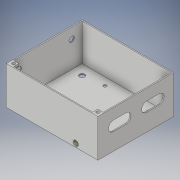
# Autodesk Inventor part: Caixa de Segurança_Sem fixação
Saved by Autodesk Inventor 2019 (Build 230136000, 136)
## iProperties
Created: 2020-05-23
Part Number: Caixa de Segurança_Sem fixação
Material: Genérico
Document SubType Name: Modeling
Designer: lukas
Density: 1 g/cm^3
Appearance: Padrão
Categories: <MemberInstance><Categories><Category DisplayName="" Mnemonic="CABLEANDHARNESS" InternalName="e4a7e005-5e42-4d16-b293-125e7f0d0512"><Category DisplayName="" Mnemonic="CONNECTORS" InternalName="6f634eba-a678-4820-a31d-2c2d5ee6728e"><CategoryParameter DisplayName="" Mnemonic="REFDES" InternalName="c3740e8c-60ab-4d5d-8584-52b73222f2f0"/><Category DisplayName="" Mnemonic="DISCRETEWIRE" InternalName="9a3407de-09b2-4cdb-8c40-9708d5144a28"/></Category></Category></Categories><FamilyTemplate><FamilyTemplateParameters></FamilyTemplateParameters></FamilyTemplate><CategoryParameterMap><ParamToTemplateMap><ParamToTemplate CategoryParameter="//CategoryParameter[@InternalName='c3740e8c-60ab-4d5d-8584-52b73222f2f0']" ConstantValue=""/></ParamToTemplateMap></CategoryParameterMap></MemberInstance>
Author: lukas
Autodesk Inventor part; units mm, degrees
ref_plane "YZ Plane" through (0, 0, 0) normal (1, 0, 0) x (0, 1, 0)
ref_plane "XZ Plane" through (0, 0, 0) normal (0, 1, 0) x (-1, 0, 0)
ref_plane "XY Plane" through (0, 0, 0) normal (0, 0, 1) x (1, 0, 0)
sketch "Esboço1" plane through (0, 0, 0) normal (0, 1, 0) x (-1, 0, 0)
  line L0 (-23.75, -30.48) -> (23.75, -30.48)
  line L1 (23.75, -30.48) -> (23.75, 30.48)
  line L2 (23.75, 30.48) -> (-23.75, 30.48)
  line L3 (-23.75, 30.48) -> (-23.75, -30.48)
  line L4 (-23.75, -30.48) -> (23.75, 30.48) construction
  line L5 (23.75, -30.48) -> (-23.75, 30.48) construction
  line L6 (-35, -35) -> (35, -35)
  line L7 (35, 35) -> (-35, 35)
  line L8 (-35, 35) -> (-35, -35)
  line L9 (-35, -35) -> (35, 35) construction
  line L10 (35, -35) -> (-35, 35) construction
  line L11 (23.75, 30.48) -> (20.75, 30.48)
  line L12 (23.75, 27.48) -> (23.75, 30.48)
  line L13 (-23.75, 30.48) -> (-20.75, 30.48)
  line L14 (-23.75, 27.48) -> (-23.75, 30.48)
  line L15 (-23.75, -30.48) -> (-20.75, -30.48)
  line L16 (-23.75, -27.48) -> (-23.75, -30.48)
  line L17 (23.75, -30.48) -> (20.75, -30.48)
  line L18 (23.75, -27.48) -> (23.75, -30.48)
  circle A0 centre (20.75, 27.48) radius 1.5
  circle A1 centre (-20.75, 27.48) radius 1.5
  circle A2 centre (-20.75, -27.48) radius 1.5
  circle A3 centre (20.75, -27.48) radius 1.5
  line L19 (35, -35) -> (50, -35)
  line L20 (50, -35) -> (50, 35)
  line L21 (50, 35) -> (35, 35)
  line L22 (50, -35) -> (40, -35)
  line L23 (40, -25) -> (40, 25)
  circle A4 centre (40, -25) radius 2.5
  circle A5 centre (40, 25) radius 2.5
  point P0 (0, 0)
  dimension "d0" = 47.5
  dimension "d1" = 60.96
  dimension "d12" = 3
  dimension "d13" = 3
  dimension "d33" = 15
  dimension "d34" = 70
  dimension "d35" = 10
  dimension "d36" = 10
  dimension "d37" = 50
  dimension "d38" = 5
  dimension "d39" = 5
  constraints: 48 end point, 6 centre point, 6 horizontal, 4 midpoint, 3 parallel, 3 perpendicular, 2 coincident, 2 point on line
  measures "d0" distance of L2.end L1.end
  measures "d1" distance of L1.end L0.end
  measures "d12" diameter of A1
  measures "d13" diameter of A2
  measures "d33" distance of L6.end L19.end
  measures "d34" distance of L19.end L20.end
  measures "d35" distance of L19.end L22.end
  measures "d36" distance of L22.end L23.start
  measures "d37" distance of L23.start L23.end
  measures "d38" diameter of A4
  measures "d39" diameter of A5
extrude "Extrusão1" add sketch "Esboço1" along normal blind 35 contours L3 L2 L1 L0 | L8 L7 L21 L20 L19 L6 | A4 | A5
shell "Casca1" thickness 1 outward yes removed faces 5 at (6.6326, 35, -8.7485) at (19.2549, 23.3333, 27.3593) at (-22.2451, 23.3333, -27.6007) at (-22.2451, 23.3333, 27.3593) at (19.2549, 23.3333, -27.6007)
sketch "Esboço3" plane through (-50, 0, -35) normal (0, 1, 0) x (1, 0, 0)
  line L0 (0, 0) -> (85, 0) projected
  line L1 (0, 0) -> (10, 0)
  line L2 (10, 0) -> (10, -10)
  line L3 (10, -10) -> (10, -60)
  circle A0 centre (10, -10) radius 2.5
  circle A1 centre (10, -60) radius 2.5
  point P0 (50, -35)
  dimension "d40" = 10
  dimension "d41" = 10
  dimension "d42" = 50
  dimension "d43" = 5
  dimension "d44" = 5
  constraints: 6 end point, 2 centre point, 2 coincident, 2 point on line, 1 vertical
  measures "d40" distance of L0.start L1.end
  measures "d41" distance of L1.end L2.end
  measures "d42" distance of L2.end L3.end
  measures "d43" diameter of A0
  measures "d44" diameter of A1
extrude "Extrusão3" cut sketch "Esboço3" against normal blind 1
sketch "Esboço4" plane through (-50, 0, -35) normal (1, 0, 0) x (0, 0, -1)
  line L0 (-70, 0) -> (-70, 35) projected
  line L1 (-70, 35) -> (-60, 35)
  line L2 (-70, 35) -> (0, 35) projected
  line L3 (-60, 35) -> (-60, 25)
  line L4 (0, 0) -> (0, 35) projected
  line L5 (0, 35) -> (-10, 35)
  line L6 (-10, 35) -> (-10, 25)
  circle A0 centre (-60, 25) radius 2.5
  circle A1 centre (-10, 25) radius 2.5
  point P0 (-35, 0)
  dimension "d47" = 10
  dimension "d48" = 10
  dimension "d49" = 10
  dimension "d50" = 10
  dimension "d51" = 5
  dimension "d52" = 5
  constraints: 8 end point, 2 centre point, 2 coincident, 2 perpendicular, 2 point on line
  measures "d47" distance of L0.end L1.end
  measures "d48" distance of L1.end L3.end
  measures "d49" distance of L2.end L5.end
  measures "d50" distance of L5.end L6.end
  measures "d51" diameter of A0
  measures "d52" diameter of A1
extrude "Extrusão4" cut sketch "Esboço4" against normal blind 1
sketch "Esboço5" plane through (0, 35, 0) normal (0, 1, 0) x (1, 0, 0)
  line L0 (-50, -35) -> (35, -35) projected
  line L1 (35, -35) -> (30, -35)
  line L2 (30, -35) -> (30, -30)
  line L3 (30, -30) -> (35, -30)
  line L4 (35, -30) -> (35, -35)
  line L5 (-50, -35) -> (-45, -35)
  line L6 (-45, -35) -> (-45, -30)
  line L7 (-45, -30) -> (-50, -30)
  line L8 (-50, -30) -> (-50, -35)
  circle A0 centre (-47.5, -32.5) radius 1.5
  circle A1 centre (32.5, -32.5) radius 1.5
  point P0 (0, 0)
  dimension "d63" = 5
  dimension "d64" = 5
  dimension "d65" = 5
  dimension "d66" = 5
  dimension "d67" = 3
  dimension "d68" = 3
  constraints: 16 end point, 4 parallel, 2 centre point, 2 horizontal, 2 perpendicular
  measures "d63" distance of L2.end L3.end
  measures "d64" distance of L1.end L2.end
  measures "d65" distance of L7.end L6.end
  measures "d66" distance of L6.end L5.end
  measures "d67" diameter of A0
  measures "d68" diameter of A1
extrude "Extrusão5" add sketch "Esboço5" against normal blind 2
thread "Rosca1" size "M5x0.8" class "6H" standard "ANSI Metric M Profile" full length
thread "Rosca2" size "M5x0.8" class "6H" standard "ANSI Metric M Profile" full length
thread "Rosca3" size "M5x0.8" class "6H" standard "ANSI Metric M Profile" full length
thread "Rosca4" size "M5x0.8" class "6H" standard "ANSI Metric M Profile" full length
sketch "Esboço9" plane through (-51, -1, 36) normal (0, 0, 1) x (1, 0, 0)
  line L0 (86, 1) -> (1, 1) projected
  line L1 (86, 1) -> (66, 1)
  line L2 (66, 1) -> (66, 3.5)
  circle A0 centre (66, 3.5) radius 2.5
  point P0 (51, 1)
  dimension "d101" = 20
  dimension "d102" = 2.5
  constraints: 4 end point, 1 coincident, 1 perpendicular, 1 point on line, 1 vertical alignment, 2 other
  measures "d101" distance of L0.start L1.end
  measures "d102" distance of L1.end L2.end
extrude "Extrusão9" cut sketch "Esboço9" against normal blind 2
sketch "Esboço10" plane through (36, -1, 36) normal (1, 0, 0) x (0, 0, -1)
  line L0 (1, 34) -> (1, 36) projected
  line L1 (1, 36) -> (1, 21)
  line L2 (1, 1) -> (1, 34) projected
  line L3 (71, 1) -> (71, 36) projected
  circle A0 centre (26.7092, 21) radius 4.65
  line L4 (26.7092, 25.65) -> (14.7092, 25.65)
  circle A1 centre (14.7092, 21) radius 4.65
  line L5 (14.7092, 16.35) -> (26.7092, 16.35)
  circle A2 centre (58.195, 21) radius 4.65
  line L6 (58.195, 25.65) -> (46.195, 25.65)
  circle A3 centre (46.195, 21) radius 4.65
  line L7 (46.195, 16.35) -> (58.195, 16.35)
  line L8 (1, 21) -> (71, 21)
  line L9 (34.7126, 21) -> (44.7126, 21)
  point P0 (36, 1)
  dimension "d105" = 15
  dimension "d107" = 9.3
  dimension "d108" = 12
  dimension "d109" = 9.3
  dimension "d110" = 12
  dimension "d111" = 10
  constraints: 14 end point, 8 point on circle, 6 tangent, 4 centre point, 4 point on line, 2 horizontal, 1 perpendicular
  measures "d105" distance of L0.end L1.end
  measures "d107" diameter of A0
  measures "d108" distance of L4.start L4.end
  measures "d109" diameter of A2
  measures "d110" distance of L6.start L6.end
  measures "d111" distance of L9.start L9.end
extrude "Extrusão10" cut sketch "Esboço10" against normal blind 2
sketch "Esboço11" plane through (-51, -1, 36) normal (0, 0, 1) x (1, 0, 0)
  circle A0 centre (66, 3.5) radius 2.5 projected
